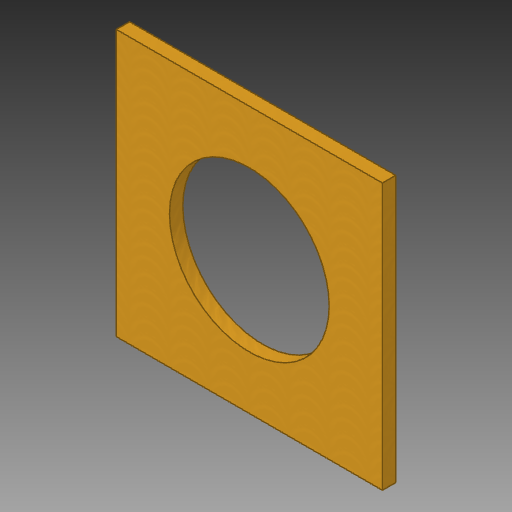
# Autodesk Inventor part: 障害物、丸１
Saved by Autodesk Inventor 2017 (Build 210142000, 142)
## iProperties
Part Number: 障害物、丸１
Material: 一般
Document SubType Name: Modeling
Designer: 雪村
Density: 1 g/cm^3
Appearance: 溶接 - 真鍮
Mass: 968.296 g
Surface Area: 1555.88 cm^2
Volume: 968.296 cm^3
Author: 雪村
Autodesk Inventor part; units mm, degrees
ref_plane "YZ Plane" through (0, 0, 0) normal (1, 0, 0) x (0, 1, 0)
ref_plane "XZ Plane" through (0, 0, 0) normal (0, 1, 0) x (-1, 0, 0)
ref_plane "XY Plane" through (0, 0, 0) normal (0, 0, 1) x (1, 0, 0)
sketch "スケッチ1" plane through (0, 0, 0) normal (0, 0, 1) x (1, 0, 0)
  line L0 (150, 150) -> (150, -150)
  line L1 (150, -150) -> (-150, -150)
  line L2 (-150, -150) -> (-150, 150)
  line L3 (-150, 150) -> (150, 150)
  circle A0 centre (0, 0) radius 90
  dimension "d0" = 300
  dimension "d1" = 180
  constraints: 8 end point, 2 coincident, 1 centre point, 1 horizontal, 9 other
  measures "d0" distance of L2.end L0.start
  measures "d1" diameter of A0
extrude "押し出し1" add sketch "スケッチ1" along normal blind 15
